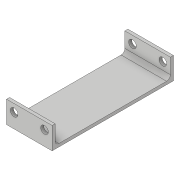
# Autodesk Inventor part: Top grip collecter grip
Saved by Autodesk Inventor 2020 (Build 240168000, 168)
## iProperties
Created: 2019-10-17
Part Number: Top grip collecter grip
Material: Generic
Document SubType Name: Modeling
Designer: ball
Density: 1 g/cm^3
Appearance: Default
Author: ball
Autodesk Inventor part; units mm, degrees
ref_plane "YZ Plane" through (0, 0, 0) normal (1, 0, 0) x (0, 1, 0)
ref_plane "XZ Plane" through (0, 0, 0) normal (0, 1, 0) x (-1, 0, 0)
ref_plane "XY Plane" through (0, 0, 0) normal (0, 0, 1) x (1, 0, 0)
sketch "Sketch1" plane through (0, 0, 0) normal (0, 1, 0) x (-1, 0, 0)
  line L0 (0, 0) -> (76.2, 0)
  line L1 (76.2, 0) -> (76.2, -203.2)
  line L2 (76.2, -203.2) -> (0, -203.2)
  line L3 (0, -203.2) -> (0, 0)
  dimension "d0" = 76.2
  dimension "d1" = 203.2
  constraints: 8 end point, 2 parallel, 1 horizontal, 1 perpendicular
  measures "d0" distance of L1.end L2.end
  measures "d1" distance of L0.end L1.end
extrude "Extrusion1" add sketch "Sketch1" along normal blind 36.83
sketch "Sketch2" plane through (-76.2, 0, 0) normal (0, 0, 1) x (1, 0, 0)
  circle A0 centre (63.5, 24.13) radius 6.4135
  circle A1 centre (12.7, 24.13) radius 6.4135
  line L0 (76.2, 0) -> (0, 0) projected
  line L1 (0, 0) -> (0, 36.83) projected
  dimension "d4" = 12.827
  dimension "d5" = 12.827
  dimension "d6" = 24.13
  dimension "d7" = 24.13
  dimension "d8" = 50.8
  dimension "d9" = 12.7
  constraints: 2 centre point
  measures "d4" diameter of A0
  measures "d5" diameter of A1
  measures "d6" distance from line of L0 A1.centre
  measures "d7" distance from line of L0 A0.centre
  measures "d8" distance of A0.centre A1.centre
  measures "d9" distance from line of L1 A1.centre
extrude "Extrusion2" cut sketch "Sketch2" against normal through all
sketch "Sketch3" plane through (0, 0, 0) normal (1, 0, 0) x (0, 0, -1)
  line L0 (0, 36.83) -> (203.2, 36.83) projected
  line L1 (5.08, 36.83) -> (198.12, 36.83)
  line L2 (198.12, 36.83) -> (198.12, 5.08)
  line L3 (198.12, 5.08) -> (5.08, 5.08)
  line L4 (5.08, 5.08) -> (5.08, 36.83)
  line L5 (0, 0) -> (0, 36.83) projected
  line L6 (203.2, 0) -> (203.2, 36.83) projected
  line L7 (203.2, 0) -> (0, 0) projected
  dimension "d12" = 5.08
  dimension "d13" = 5.08
  dimension "d14" = 5.08
  constraints: 8 end point, 2 parallel, 1 horizontal, 1 perpendicular, 1 point on line
  measures "d12" distance between parallel lines of L5 L4
  measures "d13" distance between parallel lines of L6 L2
  measures "d14" distance between parallel lines of L7 L3
extrude "Extrusion3" cut sketch "Sketch3" against normal through all contours L0 L2 L3 L4
fillet "Fillet1" radius 6.35 2 edges at (-38.1, 5.08, -198.12) (-38.1, 5.08, -5.08)
ref_plane "Work Plane1" through (-38.1, 0, 0) normal (1, 0, 0) x (0, 0, -1)
body "Solid1"
